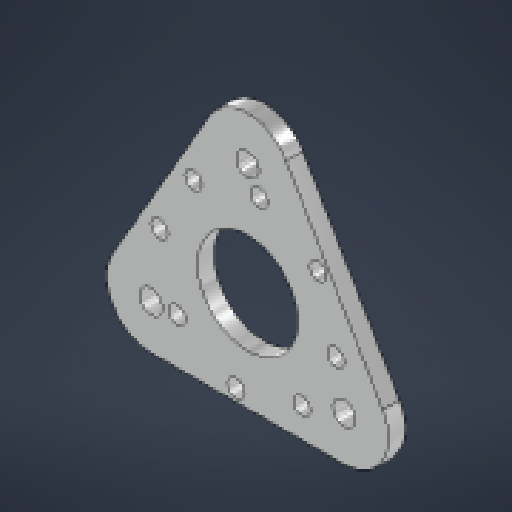
# Autodesk Inventor part: PLATE,TURRET,MOTOR,MOUNT
Saved by Autodesk Inventor 2026 (Build 300175000, 175)
## iProperties
Created: 2026-02-09
Part Number: PLATE,TURRET,MOTOR,MOUNT
Material: Aluminum 6061
Document SubType Name: Sheet Metal
Designer: littl
Density: 2.7 g/cm^3
Sheet Metal Rule: Default
Appearance: Aluminum - Flat
Author: littl
Autodesk Inventor part; units mm, degrees
ref_plane "YZ Plane" through (0, 0, 0) normal (1, 0, 0) x (0, 1, 0)
ref_plane "XZ Plane" through (0, 0, 0) normal (0, 1, 0) x (-1, 0, 0)
ref_plane "XY Plane" through (0, 0, 0) normal (0, 0, 1) x (1, 0, 0)
sketch "Sketch2" plane through (0, 0, 0) normal (0, 0, 1) x (1, 0, 0)
  line L0 (27.4963, -15.875) -> (0, 0) construction
  arc A0 (-38.4948, -9.525) -> (-27.4963, -28.575) centre (-27.4963, -15.875) ccw
  arc A1 (27.4963, -28.575) -> (38.4948, -9.525) centre (27.4963, -15.875) ccw
  arc A2 (10.9985, 38.1) -> (-10.9985, 38.1) centre (0, 31.75) ccw
  line L1 (-38.4948, -9.525) -> (-10.9985, 38.1)
  line L2 (10.9985, 38.1) -> (38.4948, -9.525)
  line L3 (27.4963, -28.575) -> (-27.4963, -28.575)
  point P0 (-25.1827, 3.3154)
  point P1 (-20.1512, -15.4625)
  point P2 (-3.3154, -25.1827)
  point P3 (15.4625, -20.1512)
  point P4 (25.1827, -3.3154)
  point P5 (20.1512, 15.4625)
  point P6 (3.3154, 25.1827)
  point P7 (-15.4625, 20.1512)
  dimension "d74" = 31.75
  dimension "d77" = 360
  dimension "d80" = 25.4
  dimension "d83" = 360
  dimension "d92" = 12.7
  constraints: 8 end point, 6 point on circle, 6 tangent, 3 centre point, 3 coincident, 2 equal radius, 1 symmetric about line, 1 vertical alignment, 13 other
  measures "d74" distance of point (0, 0) point (0, 31.75)
  measures "d80" distance of point (0, 0) point (-25.183, 3.315)
  measures "d92" radius of A1
extrude "Plate2" add sketch "Sketch2" along normal blind 4.7625
hole "Hole3" at (-27.4963, -15.875, 0) at (0, 31.75, 0) at (27.4963, -15.875, 0) direction (0, 0, 1) diameter 6.5278 end through all clearance for "Flat Head Machine Screw (82)" size "1/4" standard "Ansi Unified Screw Threads"
hole "Hole4" at (0, 0, 0) direction (0, 0, 1) diameter 28.575 end through all
hole "Hole5" at (-25.1827, 3.3154, 0) at (15.4625, -20.1512, 0) at (25.1827, -3.3154, 0) at (-15.4625, 20.1512, 0) direction (0, 0, 1) diameter 4.9784 end through all clearance for "Flat Head Machine Screw (82)" size "#10" standard "Ansi Unified Screw Threads"
equation "\"BendRadius\" = Thickness"
equation "\"BendReliefWidth\" = Thickness"
equation "\"BendReliefDepth\" = 0.5 * Thickness"
equation "\"CornerReliefSize\" = 4 * Thickness"
equation "\"MinimumRemnant\" = 2 * Thickness"
equation "\"TransitionRadius\" = BendRadius"
equation "\"JacobiRadiusSize\" = BendRadius"
equation "\"GapSize\" = Thickness"
equation "\"Thickness\" = 4.7625"
body "Solid2"
